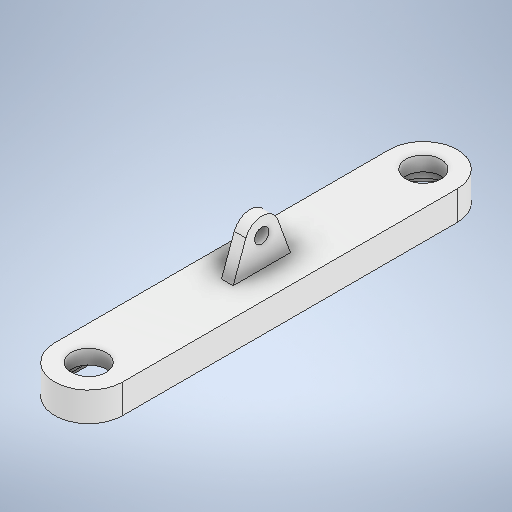
# Autodesk Inventor part: Gripper_arms
Saved by Autodesk Inventor 2025.2 (Build 292293000, 293)
## iProperties
Created: 2025-01-12
Part Number: Gripper_arms
Material: Generic
Document SubType Name: Modeling
Designer: caomi
Density: 1 g/cm^3
Appearance: Default
Author: caomi
Autodesk Inventor part; units mm, degrees
ref_plane "YZ Plane" through (0, 0, 0) normal (1, 0, 0) x (0, 1, 0)
ref_plane "XZ Plane" through (0, 0, 0) normal (0, 1, 0) x (-1, 0, 0)
ref_plane "XY Plane" through (0, 0, 0) normal (0, 0, 1) x (1, 0, 0)
sketch "Sketch1" plane through (0, 0, 0) normal (0, 1, 0) x (-1, 0, 0)
  line L0 (-7, 41.5) -> (7, 41.5)
  line L1 (7, 41.5) -> (7, -41.5)
  line L2 (7, -41.5) -> (-7, -41.5)
  line L3 (-7, -41.5) -> (-7, 41.5)
  line L4 (-7, 41.5) -> (7, -41.5) construction
  line L5 (7, 41.5) -> (-7, -41.5) construction
  circle A0 centre (0, 34.5) radius 3.6
  circle A1 centre (0, -34.5) radius 3.6
  line L6 (13.7936, 0) -> (-15.5073, 0) construction
  point P0 (0, 0)
  dimension "d0" = 7.2
  dimension "d1" = 69
  dimension "d2" = 83
  dimension "d3" = 14
  constraints: 14 end point, 2 centre point, 2 horizontal, 2 midpoint, 2 parallel, 2 vertical alignment, 1 perpendicular, 1 point on line, 1 other
  measures "d0" diameter of A0
  measures "d1" distance of A0.centre A1.centre
  measures "d2" distance of L0.end L1.end
  measures "d3" distance of L0.start L0.end
extrude "Extrusion1" add sketch "Sketch1" along normal mid plane 6
sketch "Sketch2" plane through (0, 0, 0) normal (1, 0, 0) x (0, 1, 0)
  circle A0 centre (9, 0) radius 3.5
  line L0 (10.1971, -3.2889) -> (3, -5.9084)
  line L1 (3, -41.5) -> (3, 41.5) projected
  line L2 (10.1971, 3.2889) -> (3, 5.9084)
  line L3 (9, 0) -> (-7.9221, 0) construction
  circle A1 centre (9, 0) radius 1.5
  point P0 (0, 0)
  point P1 (16.3025, 1.2439)
  point P2 (5, 7.6173)
  point P3 (5, -5.09)
  point P4 (3, 0)
  dimension "d6" = 7
  dimension "d11" = 20
  dimension "d12" = 6
  dimension "d13" = 3
  constraints: 6 end point, 2 centre point, 2 point on circle, 2 point on line, 1 horizontal, 1 horizontal alignment, 1 midpoint, 1 tangent, 1 other
  measures "d6" diameter of A0
  measures "d11" angle of L3 L2
  measures "d12" distance of point (3, 0) L3.start
  measures "d13" diameter of A1
extrude "Extrusion2" add sketch "Sketch2" along normal mid plane 2.4
fillet "Fillet1" radius 7 4 edges at (-7, 0, 41.5) (7, 0, 41.5) (-7, 0, -41.5) (7, 0, -41.5)
sketch "Sketch5" plane through (0, -3, 0) normal (0, -1, 0) x (1, 0, 0)
  arc A0 (-7, -34.5) -> (7, -34.5) centre (0, -34.5) ccw projected
  arc A1 (-7, -34.5) -> (7, -34.5) centre (0, -34.5) ccw projected
  line L0 (7, -34.5) -> (7, 34.5) projected
  arc A2 (7, 34.5) -> (-7, 34.5) centre (0, 34.5) ccw projected
  line L1 (-7, 34.5) -> (-7, -34.5) projected
  circle A3 centre (0, 34.5) radius 3.6 projected
  circle A4 centre (0, -34.5) radius 3.6 projected
  arc A5 (-5.5, -34.5) -> (5.5, -34.5) centre (0, -34.5) ccw
  line L2 (5.5, -34.5) -> (5.5, 34.5)
  arc A6 (5.5, 34.5) -> (-5.5, 34.5) centre (0, 34.5) ccw
  line L3 (-5.5, 34.5) -> (-5.5, -34.5)
  point P0 (0, 0)
  dimension "d32" = 1.5
  constraints: 4 end point, 4 point on circle, 2 centre point, 3 other
  measures "d32" distance between parallel lines of L1 L3
extrude "Extrusion5" cut sketch "Sketch5" against normal blind 3 contours L3 A6 L2 A5
sketch "Sketch7" plane through (0, 0, 0) normal (0, 0, 1) x (1, 0, 0)
  point P0 (0, 0)
sketch "Sketch8" plane through (0, 0, 0) normal (0, 0, 1) x (1, 0, 0)
  line L0 (-5.5, -2.5) -> (-6.5, -1.5)
  line L1 (-6.5, -1.5) -> (-5.5, -0.5)
  line L2 (-6.5, -1.5) -> (-5.5, -1.5) construction
  line L3 (-5.5, -3) -> (-5.5, 0) projected
  point P0 (0, 0)
  dimension "d38" = 1
  dimension "d39" = 45
  dimension "d42" = 0.5
  constraints: 7 end point, 3 point on line, 1 horizontal, 1 midpoint, 1 other
  measures "d38" distance of L0.end L2.end
  measures "d39" angle of L3 L0
  measures "d42" distance of L3.start L0.start
sketch3d "3D Sketch1"
  arc A0 (5.5, -3, -34.5) -> (3.8891, -3, -38.3891) centre (0, -3, -34.5) ccw
  arc A1 (3.8891, -3, -38.3891) -> (0, -3, -40) centre (0, -3, -34.5) ccw
  arc A2 (0, -3, -40) -> (-3.8891, -3, -38.3891) centre (0, -3, -34.5) ccw
  arc A3 (-3.8891, -3, -38.3891) -> (-5.5, -3, -34.5) centre (0, -3, -34.5) ccw
  line L0 (5.5, -3, -34.5) -> (5.5, -3, 34.5)
  arc A4 (-5.5, -3, 34.5) -> (-3.8891, -3, 38.3891) centre (0, -3, 34.5) ccw
  arc A5 (-3.8891, -3, 38.3891) -> (0, -3, 40) centre (0, -3, 34.5) ccw
  arc A6 (0, -3, 40) -> (3.8891, -3, 38.3891) centre (0, -3, 34.5) ccw
  arc A7 (3.8891, -3, 38.3891) -> (5.5, -3, 34.5) centre (0, -3, 34.5) ccw
  line L1 (-5.5, -3, 34.5) -> (-5.5, -3, -34.5)
sweep "Sweep1" cut profiles "Sketch8" path "3D Sketch1"
equation "\"d10\" = 0.5 * d3"
body "Solid1"
